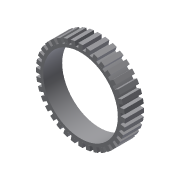
# Autodesk Inventor part: 200_Holder_Lambdaplate_1
Saved by Autodesk Inventor 2019 (Build 230136000, 136)
## iProperties
Created: 2019-07-08
Part Number: 200_Holder_Lambdaplate_1
Material: Generic
Document SubType Name: Modeling
Designer: diederichbenedict
Density: 1 g/cm^3
Appearance: Default
Author: diederichbenedict
Autodesk Inventor part; units mm, degrees
ref_plane "YZ Plane" through (0, 0, 0) normal (1, 0, 0) x (0, 1, 0)
ref_plane "XZ Plane" through (0, 0, 0) normal (0, 1, 0) x (-1, 0, 0)
ref_plane "XY Plane" through (0, 0, 0) normal (0, 0, 1) x (1, 0, 0)
sketch "Sketch6" plane through (0, 0, 0) normal (0, 0, 1) x (1, 0, 0)
  circle A0 centre (0, 0) radius 12.5 projected
  circle A1 centre (0, 0) radius 12.8
  circle A2 centre (0, 0) radius 13.8
  dimension "d32" = 0.3
  dimension "d33" = 1
  constraints: 2 centre point
  measures "d32" radial gap between concentric circles of A0 A1
  measures "d33" radial gap between concentric circles of A1 A2
ref_plane "Work Plane1" through (-12.5, -12.5, 6.5) normal (0, 0, 1) x (1, 0, 0)
extrude "Extrusion4" add sketch "Sketch6" along normal up to surface (6.5 mm away) contours A2
sketch "Sketch7" plane through (0, 0, 0) normal (0, 0, -1) x (-1, 0, 0)
  line L0 (13.8, 0) -> (0, 0)
  line L1 (0, 0) -> (0, 0)
  line L2 (0, 0) -> (13.7825, -0.7223)
  line L3 (0, 0) -> (0, 0) construction
  line L4 (0, 0) -> (0, 0) construction
  line L5 (0, 0) -> (0, 0) construction
  line L6 (13.7825, -0.7223) -> (15.2804, -0.8008) construction
  line L7 (15.2804, -0.7223) -> (15.2804, 0)
  arc A0 (13.7825, -0.7223) -> (13.8, 0) centre (-1.1, 0) ccw
  line L8 (15.2804, 0) -> (13.8, 0)
  line L9 (13.7825, -0.7223) -> (15.2804, -0.7223)
  circle A1 centre (0, 0) radius 13.8 construction
  line L10 (13.7825, 0.7223) -> (15.2804, 0.8008) construction
  line L11 (15.2804, 0.7223) -> (15.2804, 0)
  arc A2 (13.8, 0) -> (13.7825, 0.7223) centre (-1.1, 0) ccw
  line L12 (13.7825, 0.7223) -> (15.2804, 0.7223)
  dimension "d37" = 0
  dimension "d38" = 1.5
  dimension "d44" = 3
  constraints: 26 end point, 4 point on circle, 3 perpendicular, 3 symmetric about line, 2 centre point, 2 collinear, 2 horizontal, 1 equal length, 1 midpoint, 1 vertical, 3 other
  measures "d37" distance between parallel lines of L4 L2
  measures "d38" distance of L2.end L6.end
  measures "d44" angle of L0 L2
extrude "Extrusion5" add sketch "Sketch7" against normal up to surface (6.5 mm away) contours L8 L7 L9 A0 | A2 L12 L11 L8
pattern_circular "Circular Pattern2" count 36 over 360 about axis through (0, 0, 0) along (0, 0, 1) of "Extrusion5"
body "Solid2"
